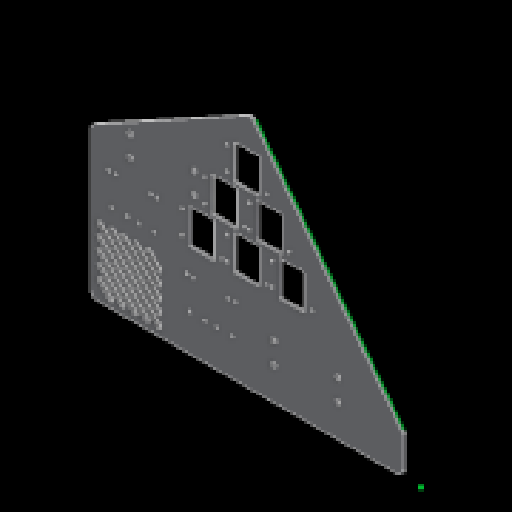
# Autodesk Inventor part: SideChestPanel
Saved by Autodesk Inventor 2025.2 (Build 292293000, 293)
## iProperties
Created: 2025-10-06
Part Number: SideChestPanel
Material: Generic
Document SubType Name: Sheet Metal
Designer: valer
Density: 1 g/cm^3
Sheet Metal Rule: Default
Appearance: Default
Author: valer
Autodesk Inventor part; units mm, degrees
note: some values were not read from the file. Chosen so that the rebuilt part matches the saved one: edges of "OutsideFilletsFeature".
ref_plane "YZ Plane" through (0, 0, 0) normal (1, 0, 0) x (0, 1, 0)
ref_plane "XZ Plane" through (0, 0, 0) normal (0, 1, 0) x (-1, 0, 0)
ref_plane "XY Plane" through (0, 0, 0) normal (0, 0, 1) x (1, 0, 0)
sketch "Base" plane through (0, 0, 0) normal (0, 0, 1) x (1, 0, 0)
  line L0 (-378.7052, 89.8796) -> (-378.7052, 174.3855)
  line L1 (-378.7052, 174.3855) -> (-195.1416, 275.4647)
  line L2 (-195.1416, 275.4647) -> (-175.6395, 271.0298)
  line L3 (-175.6395, 271.0298) -> (-18.7052, 51.3218)
  line L4 (-18.7052, 51.3218) -> (-18.7052, 2.2456)
  line L5 (-18.7052, 2.2456) -> (-378.7052, 2.2456)
  line L6 (-378.7052, 2.2456) -> (-378.7052, 89.8796)
  line L7 (-389.1847, 101.2829) -> (-389.1847, 49.3817) construction
  line L8 (-169.8355, 262.9042) -> (-11.397, 41.0903) construction
  line L9 (-372.782, 2.2456) -> (-8.9217, 2.2456) construction
  line L10 (-202.0962, 271.6351) -> (-397.656, 163.9503) construction
  point P0 (0, 0)
  dimension "d40" = 360
  dimension "d41" = 270
  dimension "d42" = 20
  dimension "d43" = 138.349
  dimension "d44" = 138.349
  measures "d40" distance of L4.end L5.end
  measures "d41" distance of L2.end L3.end
  measures "d42" distance of L1.end L2.end
  measures "d43" angle of L3 L2
  measures "d44" angle of L2 L1
extrude "Plate1" add sketch "Base" along normal blind 3
fillet "OutsideFilletsFeature" radius 6 5 edges at (-378.7052, 2.2456, 1.5) (-18.7052, 2.2456, 1.5) (-18.7052, 51.3218, 1.5) (-175.6395, 271.0298, 1.5) (-195.1416, 275.4647, 1.5)
sketch "HardwareMountHoles" plane through (0, 0, 0) normal (0, 0, -1) x (-1, 0, 0)
  circle A0 centre (175.3952, 206.6354) radius 1.5 projected
  circle A1 centre (221.3566, 233.1714) radius 1.5 projected
  circle A2 centre (149.4146, 161.6352) radius 1.5 projected
  circle A3 centre (195.3761, 161.6353) radius 1.5 projected
  circle A4 centre (195.3761, 188.1712) radius 1.5 projected
  circle A5 centre (221.3567, 206.6355) radius 1.5 projected
  circle A6 centre (201.3761, 161.6355) radius 1.5
  circle A7 centre (247.3376, 161.6357) radius 1.5
  circle A8 centre (247.3375, 188.1716) radius 1.5
  circle A9 centre (227.3571, 116.6357) radius 1.5
  circle A10 centre (273.3186, 116.6361) radius 1.5
  circle A11 centre (273.3184, 143.172) radius 1.5
  circle A12 centre (175.3956, 116.6353) radius 1.5
  circle A13 centre (221.3571, 116.6356) radius 1.5
  circle A14 centre (221.3569, 143.1715) radius 1.5
  circle A15 centre (123.4341, 116.635) radius 1.5
  circle A16 centre (169.3956, 116.6352) radius 1.5
  circle A17 centre (169.3954, 143.1711) radius 1.5
  circle A18 centre (123.4339, 143.1709) radius 1.5
  point P0 (0, 0)
  constraints: 13 centre point, 26 other
extrude "HardwareMountHolesFeature" cut sketch "HardwareMountHoles" against normal blind 3 contours A0 | A1 | A2 | A3 | A4 | A5 | A6 | A7 | A8 | A9 | A10 | A11 | A12 | A13 | A14 | A15 | A16 | A17
sketch "HeatsinkCut1" plane through (0, 0, 3) normal (0, 0, 1) x (1, 0, 0)
  line L0 (-185.8757, 238.2531) -> (-210.9757, 238.2534) projected
  line L1 (-185.876, 201.5531) -> (-185.8757, 238.2531) projected
  line L2 (-210.9757, 238.2534) -> (-210.976, 201.5534) projected
  line L3 (-210.976, 201.5534) -> (-185.876, 201.5531) projected
  point P0 (0, 0)
extrude "HeatsinkCut1Feature" cut sketch "HeatsinkCut1" against normal blind 3
sketch "HeatsinkCut2" plane through (0, 0, 3) normal (0, 0, 1) x (1, 0, 0)
  line L0 (-159.8953, 193.2532) -> (-184.9953, 193.2533) projected
  line L1 (-184.9953, 193.2533) -> (-184.9954, 156.5533) projected
  line L2 (-159.8954, 156.5532) -> (-159.8953, 193.2532) projected
  line L3 (-184.9954, 156.5533) -> (-159.8954, 156.5532) projected
  point P0 (0, 0)
extrude "HeatsinkCut2Feature" cut sketch "HeatsinkCut2" against normal blind 3
sketch "HeatsinkCut3" plane through (0, 0, 3) normal (0, 0, 1) x (1, 0, 0)
  line L0 (-211.8568, 193.2535) -> (-236.9568, 193.2536) projected
  line L1 (-211.8569, 156.5535) -> (-211.8568, 193.2535) projected
  line L2 (-236.9569, 156.5536) -> (-211.8569, 156.5535) projected
  line L3 (-236.9569, 156.5536) -> (-236.9568, 193.2536)
  point P0 (0, 0)
  constraints: 2 end point
extrude "HeatsinkCut3Feature" cut sketch "HeatsinkCut3" against normal blind 3
sketch "HeatsinkCut4" plane through (0, 0, 3) normal (0, 0, 1) x (1, 0, 0)
  line L0 (-237.8376, 148.2538) -> (-262.9376, 148.254) projected
  line L1 (-262.9376, 148.254) -> (-262.9379, 111.554) projected
  line L2 (-237.8379, 111.5538) -> (-237.8376, 148.2538) projected
  line L3 (-262.9379, 111.554) -> (-237.8379, 111.5538) projected
  point P0 (0, 0)
extrude "HeatsinkCut4Feature" cut sketch "HeatsinkCut4" against normal blind 3
sketch "HeatsinkCut5" plane through (0, 0, 3) normal (0, 0, 1) x (1, 0, 0)
  line L0 (-185.8761, 148.2534) -> (-210.9761, 148.2535) projected
  line L1 (-185.8764, 111.5534) -> (-185.8761, 148.2534) projected
  line L2 (-210.9764, 111.5535) -> (-185.8764, 111.5534) projected
  line L3 (-210.9761, 148.2535) -> (-210.9764, 111.5535) projected
  line L4 (-185.8761, 148.2534) -> (-210.9761, 148.2535) projected
  point P0 (0, 0)
extrude "HeatsinkCut5Feature" cut sketch "HeatsinkCut5" against normal blind 3
sketch "HeatsinkCut6" plane through (0, 0, 3) normal (0, 0, 1) x (1, 0, 0)
  line L0 (-133.9147, 148.253) -> (-159.0147, 148.2532) projected
  line L1 (-133.9148, 111.553) -> (-133.9147, 148.253) projected
  line L2 (-159.0147, 148.2532) -> (-159.0148, 111.5532) projected
  line L3 (-133.9147, 148.253) -> (-159.0147, 148.2532) projected
  line L4 (-159.0147, 148.2532) -> (-159.0148, 111.5532) projected
  line L5 (-159.0148, 111.5532) -> (-133.9148, 111.553) projected
  point P0 (0, 0)
extrude "HeatsinkCut6Feature" cut sketch "HeatsinkCut6" against normal blind 3
sketch "AdjustToProduction" plane through (0, 0, 3) normal (0, 0, 1) x (1, 0, 0)
  line L0 (-18.7052, 49.399) -> (-18.7052, 8.2456) projected
  line L1 (-18.7052, 46.0604) -> (-192.9162, 274.9586)
  line L2 (-174.313, 269.1727) -> (-19.8228, 52.8864) projected
  line L3 (-192.9162, 274.9586) -> (-177.8649, 271.5359) projected
  arc A0 (-174.313, 269.1727) -> (-177.8649, 271.5359) centre (-179.1954, 265.6852) ccw projected
  arc A1 (-18.7052, 49.399) -> (-19.8228, 52.8864) centre (-24.7052, 49.399) ccw projected
  point P0 (0, 0)
  constraints: 2 end point, 1 point on line
extrude "AdjustToProductionFeature" cut sketch "AdjustToProduction" against normal blind 3
delete faces "Delete1" heal yes whole lump no faces at (-196.2577, 274.7609, 1)
fillet "ProductionReFilletFeature" radius 6 3 edges at (-193.8448, 276.1787, 1.5) (-18.7052, 46.0604, 1.5) (-378.7052, 174.3855, 1.5)
sketch "WidenHeatsinkHoles" plane through (-372.7052, 2.2456, 3) normal (0, 0, 1) x (1, 0, 0)
  arc A0 (354, 41.7913) -> (352.7745, 45.425) centre (348, 41.7913) ccw projected
  line L0 (352.7745, 45.425) -> (181.995, 269.8145) projected
  arc A1 (181.995, 269.8145) -> (174.3264, 271.4366) centre (177.2206, 266.1807) ccw projected
  line L1 (-2.8941, 173.8502) -> (174.3264, 271.4366) projected
  line L2 (-6, 6) -> (-6, 168.5943) projected
  arc A2 (-6, 6) -> (0, 0) centre (0, 6) ccw projected
  line L3 (348, 0) -> (0, 0) projected
  arc A3 (348, 0) -> (354, 6) centre (348, 6) ccw projected
  line L4 (354, 41.7913) -> (354, 6) projected
  circle A4 centre (145.3481, 114.3902) radius 1.5 projected
  circle A5 centre (249.2711, 114.3895) radius 1.5 projected
  circle A6 centre (99.3868, 140.9265) radius 1.5 projected
  circle A7 centre (171.329, 159.39) radius 1.5 projected
  circle A8 centre (151.3485, 204.3899) radius 1.5 projected
  circle A9 centre (197.31, 204.3898) radius 1.5 projected
  circle A10 centre (151.3483, 140.926) radius 1.5 projected
  circle A11 centre (99.3866, 114.3906) radius 1.5 projected
  circle A12 centre (203.3096, 114.3897) radius 1.5 projected
  circle A13 centre (151.3481, 114.39) radius 1.5 projected
  circle A14 centre (223.2906, 159.3897) radius 1.5 projected
  circle A15 centre (125.3675, 159.3902) radius 1.5 projected
  circle A16 centre (177.3291, 159.3898) radius 1.5 projected
  circle A17 centre (151.3485, 230.9258) radius 1.5 projected
  circle A18 centre (177.3291, 185.9257) radius 1.5 projected
  circle A19 centre (125.3677, 185.9261) radius 1.5 projected
  circle A20 centre (203.3098, 140.9256) radius 1.5 projected
  circle A21 centre (197.3096, 114.3897) radius 1.5 projected
  line L5 (186.8292, 199.3076) -> (161.7292, 199.3078) projected
  line L6 (161.7292, 199.3078) -> (161.7295, 236.0078) projected
  line L7 (161.7295, 236.0078) -> (186.8295, 236.0076) projected
  line L8 (186.8295, 236.0076) -> (186.8292, 199.3076) projected
  line L9 (212.8098, 154.3077) -> (187.7098, 154.3077) projected
  line L10 (187.7098, 154.3077) -> (187.7099, 191.0077) projected
  line L11 (187.7099, 191.0077) -> (212.8099, 191.0077) projected
  line L12 (212.8099, 191.0077) -> (212.8098, 154.3077) projected
  line L13 (135.7484, 191.0081) -> (160.8484, 191.008) projected
  line L14 (160.8484, 191.008) -> (160.8483, 154.308) projected
  line L15 (160.8483, 154.308) -> (135.7483, 154.3081) projected
  line L16 (135.7483, 154.3081) -> (135.7484, 191.0081) projected
  line L17 (134.8673, 109.3082) -> (109.7673, 109.3084) projected
  line L18 (109.7673, 109.3084) -> (109.7676, 146.0084) projected
  line L19 (109.7676, 146.0084) -> (134.8676, 146.0082) projected
  line L20 (134.8676, 146.0082) -> (134.8673, 109.3082) projected
  line L21 (161.7288, 109.308) -> (161.7291, 146.008) projected
  line L22 (161.7291, 146.008) -> (186.8291, 146.0078) projected
  line L23 (186.8291, 146.0078) -> (186.8288, 109.3078) projected
  line L24 (186.8288, 109.3078) -> (161.7288, 109.308) projected
  line L25 (213.6904, 109.3076) -> (213.6905, 146.0076) projected
  line L26 (213.6905, 146.0076) -> (238.7905, 146.0075) projected
  line L27 (238.7905, 146.0075) -> (238.7904, 109.3075) projected
  line L28 (238.7904, 109.3075) -> (213.6904, 109.3076) projected
  line L29 (211.6904, 107.3076) -> (211.6905, 148.0076)
  line L30 (211.6905, 148.0076) -> (240.7905, 148.0075)
  line L31 (240.7905, 148.0075) -> (240.7904, 107.3075)
  line L32 (240.7904, 107.3075) -> (211.6904, 107.3076)
  line L33 (159.7288, 107.308) -> (159.7291, 148.008)
  line L34 (159.7291, 148.008) -> (188.8291, 148.0078)
  line L35 (188.8291, 148.0078) -> (188.8288, 107.3078)
  line L36 (188.8288, 107.3078) -> (159.7288, 107.308)
  line L37 (185.7098, 152.3077) -> (214.8098, 152.3077)
  line L38 (214.8098, 152.3077) -> (214.8099, 193.0077)
  line L39 (214.8099, 193.0077) -> (185.7099, 193.0077)
  line L40 (185.7099, 193.0077) -> (185.7098, 152.3077)
  line L41 (133.7483, 152.3081) -> (162.8483, 152.308)
  line L42 (162.8483, 152.308) -> (162.8484, 193.008)
  line L43 (162.8484, 193.008) -> (133.7484, 193.0081)
  line L44 (133.7484, 193.0081) -> (133.7483, 152.3081)
  line L45 (159.7292, 197.3078) -> (188.8292, 197.3076)
  line L46 (188.8292, 197.3076) -> (188.8295, 238.0076)
  line L47 (188.8295, 238.0076) -> (159.7295, 238.0078)
  line L48 (159.7295, 238.0078) -> (159.7292, 197.3078)
  line L49 (107.7673, 107.3085) -> (136.8673, 107.3082)
  line L50 (136.8673, 107.3082) -> (136.8676, 148.0082)
  line L51 (136.8676, 148.0082) -> (107.7676, 148.0085)
  line L52 (107.7676, 148.0085) -> (107.7673, 107.3085)
  arc A22 (-2.8941, 173.8502) -> (-6, 168.5943) centre (0, 168.5943) ccw projected
  point P0 (372.7052, -2.2456)
  dimension "d56" = 2
  dimension "d57" = 2
  dimension "d58" = 2
  dimension "d59" = 2
  dimension "d60" = 2
  dimension "d61" = 2
  constraints: 48 end point, 18 other
  measures "d56" distance between parallel lines of L28 L32
  measures "d57" distance between parallel lines of L24 L36
  measures "d58" distance between parallel lines of L9 L37
  measures "d59" distance between parallel lines of L15 L41
  measures "d60" distance between parallel lines of L5 L45
  measures "d61" distance between parallel lines of L17 L49
extrude "WidenHeatsinkHolesFeature" cut sketch "WidenHeatsinkHoles" against normal blind 3 contours L5 L6 L7 L8 | L9 L10 L11 L12 | L13 L14 L15 L16 | L17 L18 L19 L20 | L21 L22 L23 L24 | L25 L26 L27 L28 | L29 L30 L31 L32 | L33 L34 L35 L36 | L40 L39 L38 L37 | L44 L43 L42 L41 | L48 L47 L46 L45 | L52 L51 L50 L49
fillet "HeatsinkHoleFilletsFeature" radius 1 24 edges at (-264.9379, 109.554, 1.5) (-235.8379, 109.5538, 1.5) (-235.8376, 150.2538, 1.5) (-264.9376, 150.254, 1.5) (-212.9764, 109.5535, 1.5) (-183.8764, 109.5533, 1.5) (-183.8761, 150.2533, 1.5) (-212.9761, 150.2535, 1.5) (-209.8569, 154.5535, 1.5) (-238.9569, 154.5537, 1.5) (-238.9568, 195.2537, 1.5) (-209.8568, 195.2535, 1.5) (-186.9954, 154.5533, 1.5) (-157.8954, 154.5532, 1.5) (-186.9953, 195.2533, 1.5) (-157.8953, 195.2532, 1.5) (-161.0148, 109.5532, 1.5) (-131.9148, 109.553, 1.5) (-131.9147, 150.253, 1.5) (-161.0147, 150.2532, 1.5) (-212.976, 199.5534, 1.5) (-183.876, 199.5531, 1.5) (-183.8757, 240.2531, 1.5) (-212.9757, 240.2534, 1.5)
sketch "MountHoles1" plane through (-24.7052, 2.2456, 0) normal (0, 0, -1) x (-1, 0, 0)
  circle A0 centre (68.5, 38) radius 3
  circle A1 centre (68.5, 62) radius 3
  circle A2 centre (142.5, 62) radius 3
  circle A3 centre (142.5, 38) radius 3
  circle A4 centre (190.5, 42.5) radius 1.6
  circle A5 centre (222, 42.5) radius 1.6
  circle A6 centre (235.5, 78.42) radius 1.6
  circle A7 centre (187.0915, 78.5) radius 1.6
  circle A8 centre (308.6323, 185.9084) radius 3
  circle A9 centre (308.6324, 161.9084) radius 3
  circle A10 centre (234.6323, 185.9081) radius 3
  circle A11 centre (234.6324, 161.9081) radius 3
  circle A12 centre (311.8137, 101.5) radius 1.6
  circle A13 centre (280.3137, 101.5) radius 1.6
  circle A14 centre (276.9052, 137.5) radius 1.6
  circle A15 centre (325.3137, 137.42) radius 1.6
  point P0 (-24.7052, -2.2456)
  point P1 (300.7283, 191.2583)
  constraints: 16 centre point, 33 other
extrude "MountHoles1Feature" cut sketch "MountHoles1" against normal blind 3
sketch "MountHoles2" plane through (-372.7052, 2.2456, 3) normal (0, 0, 1) x (1, 0, 0)
  circle A0 centre (139.5, 42.5) radius 1.6
  circle A1 centre (108, 42.5) radius 1.6
  circle A2 centre (104.5915, 78.5) radius 1.6
  circle A3 centre (153, 78.42) radius 1.6
  circle A4 centre (49.6863, 101.5) radius 1.6
  circle A5 centre (18.1863, 101.5) radius 1.6
  circle A6 centre (14.7778, 137.5) radius 1.6
  circle A7 centre (63.1863, 137.42) radius 1.6
  point P0 (372.7052, -2.2456)
  constraints: 8 centre point, 16 other
extrude "MountHoles2Feature" cut sketch "MountHoles2" against normal blind 3
sketch "FrontVentHoles" plane through (-24.7052, 2.2456, 0) normal (0, 0, -1) x (-1, 0, 0)
  line L0 (344, 10) -> (269, 10) construction
  line L1 (269, 10) -> (269, 79) construction
  line L2 (269, 79) -> (344, 79) construction
  line L3 (344, 79) -> (344, 10) construction
  line L4 (348, 0) -> (0, 0) projected
  line L5 (354, 168.5943) -> (354, 6) projected
  line L6 (259, 82.5) -> (259, 32.5) construction
  line L7 (346.3137, 89) -> (263.8137, 89) construction
  line L8 (344, 22.7279) -> (331.2721, 10) construction
  line L9 (341.8787, 24.8492) -> (329.1508, 12.1213)
  line L10 (333.3934, 7.8787) -> (346.1213, 20.6066)
  arc A0 (346.1213, 20.6066) -> (341.8787, 24.8492) centre (344, 22.7279) ccw
  arc A1 (329.1508, 12.1213) -> (333.3934, 7.8787) centre (331.2721, 10) ccw
  line L11 (344, 36.8701) -> (317.1299, 10) construction
  line L12 (346.1213, 34.7487) -> (319.2513, 7.8787)
  line L13 (315.0086, 12.1213) -> (341.8787, 38.9914)
  arc A2 (346.1213, 34.7487) -> (341.8787, 38.9914) centre (344, 36.8701) ccw
  arc A3 (315.0086, 12.1213) -> (319.2513, 7.8787) centre (317.1299, 10) ccw
  line L14 (344, 51.0122) -> (302.9878, 10) construction
  line L15 (346.1213, 48.8909) -> (305.1091, 7.8787)
  line L16 (300.8665, 12.1213) -> (341.8787, 53.1335)
  arc A4 (346.1213, 48.8909) -> (341.8787, 53.1335) centre (344, 51.0122) ccw
  arc A5 (300.8665, 12.1213) -> (305.1091, 7.8787) centre (302.9878, 10) ccw
  line L17 (344, 65.1543) -> (288.8457, 10) construction
  line L18 (346.1213, 63.033) -> (290.967, 7.8787)
  line L19 (286.7244, 12.1213) -> (341.8787, 67.2756)
  arc A6 (346.1213, 63.033) -> (341.8787, 67.2756) centre (344, 65.1543) ccw
  arc A7 (286.7244, 12.1213) -> (290.967, 7.8787) centre (288.8457, 10) ccw
  line L20 (274.7035, 10) -> (343.7035, 79) construction
  line L21 (272.5822, 12.1213) -> (341.5822, 81.1213)
  line L22 (345.8249, 76.8787) -> (276.8249, 7.8787)
  arc A8 (272.5822, 12.1213) -> (276.8249, 7.8787) centre (274.7035, 10) ccw
  arc A9 (345.8249, 76.8787) -> (341.5822, 81.1213) centre (343.7035, 79) ccw
  line L23 (343.7035, 79.2965) -> (274.7035, 79.2965) construction
  line L24 (289.5528, 77.1751) -> (276.8249, 64.4472)
  line L25 (272.5822, 68.6899) -> (285.3101, 81.4178)
  arc A10 (289.5528, 77.1751) -> (285.3101, 81.4178) centre (287.4315, 79.2965) ccw
  arc A11 (272.5822, 68.6899) -> (276.8249, 64.4472) centre (274.7035, 66.5685) ccw
  line L26 (299.4523, 81.4178) -> (272.5822, 54.5477)
  line L27 (276.8249, 50.3051) -> (303.6949, 77.1751)
  arc A12 (303.6949, 77.1751) -> (299.4523, 81.4178) centre (301.5736, 79.2965) ccw
  arc A13 (272.5822, 54.5477) -> (276.8249, 50.3051) centre (274.7035, 52.4264) ccw
  line L28 (313.5944, 81.4178) -> (272.5822, 40.4056)
  line L29 (276.8249, 36.163) -> (317.837, 77.1751)
  arc A14 (317.837, 77.1751) -> (313.5944, 81.4178) centre (315.7157, 79.2965) ccw
  arc A15 (272.5822, 40.4056) -> (276.8249, 36.163) centre (274.7035, 38.2843) ccw
  line L30 (329.8579, 79.2965) -> (274.7035, 24.1421) construction
  line L31 (327.7365, 81.4178) -> (272.5822, 26.2635)
  line L32 (276.8249, 22.0208) -> (331.9792, 77.1751)
  arc A16 (331.9792, 77.1751) -> (327.7365, 81.4178) centre (329.8579, 79.2965) ccw
  arc A17 (272.5822, 26.2635) -> (276.8249, 22.0208) centre (274.7035, 24.1421) ccw
  point P0 (-24.7052, -2.2456)
  point P1 (337.636, 16.364)
  point P2 (330.565, 23.435)
  point P3 (323.4939, 30.5061)
  point P4 (316.4228, 37.5772)
  point P5 (309.2035, 44.5)
  dimension "d86" = 10
  dimension "d87" = 10
  dimension "d88" = 10
  dimension "d89" = 10
  dimension "d90" = 3
  dimension "d91" = 45
  dimension "d92" = 18
  dimension "d93" = 10
  dimension "d94" = 10
  dimension "d95" = 10
  dimension "d96" = 10
  constraints: 74 end point, 36 point on circle, 26 symmetric about line, 20 tangent, 18 centre point, 14 point on line, 11 parallel, 5 midpoint, 4 equal radius, 2 horizontal, 1 perpendicular, 1 vertical, 12 other
  measures "d86" distance between parallel lines of L4 L0
  measures "d87" distance between parallel lines of L5 L3
  measures "d88" distance between parallel lines of L6 L1
  measures "d89" distance between parallel lines of L7 L2
  measures "d90" radius of A1
  measures "d91" angle of L0 L8
  measures "d92" distance of L8.start L8.end
  measures "d93" distance between parallel lines of L11 L8
  measures "d94" distance between parallel lines of L14 L11
  measures "d95" distance between parallel lines of L17 L14
  measures "d96" distance between parallel lines of L20 L17
extrude "FrontVentHolesFeature" cut sketch "FrontVentHoles" against normal blind 3
sketch "BackVentHoles" plane through (-24.7052, 2.2456, 0) normal (0, 0, -1) x (-1, 0, 0)
  line L0 (58.5, 10) -> (4, 10) construction
  line L1 (4, 10) -> (4, 40.4422) construction
  line L2 (4, 40.4422) -> (58.5, 112.0505) construction
  line L3 (58.5, 112.0505) -> (58.5, 10) construction
  line L4 (348, 0) -> (0, 0) projected
  line L5 (166.005, 269.8145) -> (-4.7745, 45.425) projected
  line L6 (-6, 6) -> (-6, 41.7913) projected
  circle A0 centre (68.5, 38) radius 3 projected
  line L7 (8.2426, 10) -> (4, 14.2426) construction
  line L8 (6.1213, 7.8787) -> (1.8787, 12.1213)
  line L9 (6.1213, 16.364) -> (10.364, 12.1213)
  arc A1 (6.1213, 7.8787) -> (10.364, 12.1213) centre (8.2426, 10) ccw
  arc A2 (6.1213, 16.364) -> (1.8787, 12.1213) centre (4, 14.2426) ccw
  line L10 (22.3848, 10) -> (4, 28.3848) construction
  line L11 (20.2635, 7.8787) -> (1.8787, 26.2635)
  line L12 (6.1213, 30.5061) -> (24.5061, 12.1213)
  arc A3 (20.2635, 7.8787) -> (24.5061, 12.1213) centre (22.3848, 10) ccw
  arc A4 (6.1213, 30.5061) -> (1.8787, 26.2635) centre (4, 28.3848) ccw
  line L13 (4.9009, 41.626) -> (36.5269, 10) construction
  line L14 (7.0223, 43.7473) -> (38.6482, 12.1213)
  line L15 (34.4056, 7.8787) -> (2.7796, 39.5047)
  arc A5 (7.0223, 43.7473) -> (2.7796, 39.5047) centre (4.9009, 41.626) ccw
  arc A6 (34.4056, 7.8787) -> (38.6482, 12.1213) centre (36.5269, 10) ccw
  arc A7 (272.5822, 12.1213) -> (276.8249, 7.8787) centre (274.7035, 10) ccw projected
  line L16 (50.669, 10) -> (11.0127, 49.6563) construction
  line L17 (52.7904, 12.1213) -> (13.134, 51.7777)
  line L18 (8.8914, 47.535) -> (48.5477, 7.8787)
  arc A8 (48.5477, 7.8787) -> (52.7904, 12.1213) centre (50.669, 10) ccw
  arc A9 (13.134, 51.7777) -> (8.8914, 47.535) centre (11.0127, 49.6563) ccw
  line L19 (58.5, 16.3112) -> (17.1245, 57.6867) construction
  line L20 (56.3787, 14.1899) -> (15.0032, 55.5654)
  line L21 (19.2458, 59.808) -> (60.6213, 18.4325)
  arc A10 (56.3787, 14.1899) -> (60.6213, 18.4325) centre (58.5, 16.3112) ccw
  arc A11 (19.2458, 59.808) -> (15.0032, 55.5654) centre (17.1245, 57.6867) ccw
  point P0 (-24.7052, -2.2456)
  point P1 (6.1213, 12.1213)
  point P2 (13.1924, 19.1924)
  point P3 (20.7139, 25.813)
  point P4 (30.8409, 29.8282)
  point P5 (37.8122, 36.9989)
  dimension "d99" = 10
  dimension "d100" = 10
  dimension "d101" = 10
  dimension "d102" = 10
  dimension "d103" = 45
  dimension "d104" = 10
  dimension "d105" = 10
  dimension "d106" = 6
  dimension "d107" = 10
  dimension "d108" = 10
  constraints: 48 end point, 20 point on circle, 20 tangent, 11 parallel, 10 centre point, 10 point on line, 5 equal radius, 5 midpoint, 2 perpendicular, 1 horizontal
  measures "d99" distance between parallel lines of L4 L0
  measures "d100" distance between parallel lines of L6 L1
  measures "d101" distance between parallel lines of L5 L2
  measures "d102" distance from line of A0.centre L3
  measures "d103" angle of L0 L7
  measures "d104" distance between parallel lines of L10 L7
  measures "d105" distance between parallel lines of L13 L10
  measures "d106" distance of L7.start L7.end
  measures "d107" distance between parallel lines of L16 L13
  measures "d108" distance between parallel lines of L19 L16
extrude "BackVentHolesFeature" cut sketch "BackVentHoles" against normal blind 3 contours L8 A2 L9 A1 | L11 A4 L12 A3 | L14 A6 L15 A5 | A8 L18 A9 L17 | L20 A11 L21 A10
sketch "ArmBoardVents" plane through (-24.7052, 2.2456, 0) normal (0, 0, -1) x (-1, 0, 0)
  line L0 (282.7778, 109) -> (266.7778, 130)
  line L1 (266.7778, 130) -> (298.7778, 130)
  line L2 (298.7778, 130) -> (282.7778, 109)
  line L3 (289.0637, 109) -> (305.0637, 130)
  line L4 (305.0637, 130) -> (321.0637, 109)
  line L5 (321.0637, 109) -> (289.0637, 109)
  line L6 (346.3137, 89) -> (263.8137, 89) construction
  line L7 (263.8137, 144) -> (346.3137, 144) construction
  line L8 (305.0637, 89) -> (305.0637, 144) construction
  line L9 (289.0637, 109) -> (282.7778, 109) construction
  line L10 (305.0637, 130) -> (298.7778, 130) construction
  circle A0 centre (276.9052, 137.5) radius 1.6 projected
  circle A1 centre (280.3137, 101.5) radius 1.6 projected
  line L11 (327.3496, 109) -> (343.3496, 130)
  line L12 (343.3496, 130) -> (311.3496, 130)
  line L13 (311.3496, 130) -> (327.3496, 109)
  line L14 (256.5, 30) -> (174, 30) construction
  line L15 (174, 85) -> (256.5, 85) construction
  line L16 (215.25, 30) -> (215.25, 85) construction
  line L17 (231.25, 50) -> (199.25, 50)
  line L18 (199.25, 50) -> (215.25, 71)
  line L19 (231.25, 50) -> (215.25, 71)
  line L20 (208.9641, 71) -> (192.9641, 50)
  line L21 (192.9641, 50) -> (176.9641, 71)
  line L22 (176.9641, 71) -> (208.9641, 71)
  line L23 (215.25, 71) -> (208.9641, 71) construction
  line L24 (199.25, 50) -> (192.9641, 50) construction
  line L25 (221.5359, 71) -> (237.5359, 50)
  line L26 (237.5359, 50) -> (253.5359, 71)
  line L27 (253.5359, 71) -> (221.5359, 71)
  point P0 (-24.7052, -2.2456)
  point P1 (305.0637, 109)
  dimension "d111" = 32
  dimension "d112" = 5
  dimension "d113" = 14
  dimension "d114" = 7.5
  dimension "d115" = 7.5
  dimension "d116" = 14
  dimension "d117" = 20
  dimension "d118" = 20
  dimension "d119" = 5
  constraints: 56 end point, 9 horizontal, 6 symmetric about line, 5 equal length, 5 midpoint, 3 point on line, 2 collinear, 1 parallel, 1 perpendicular, 8 other
  measures "d111" distance of L0.end L1.end
  measures "d112" distance between parallel lines of L2 L3
  measures "d113" distance between parallel lines of L7 L1
  measures "d114" distance from line of A0.centre L1
  measures "d115" distance from line of L9 A1.centre
  measures "d116" distance from line of L15 L18.end
  measures "d117" distance between parallel lines of L6 L5
  measures "d118" distance between parallel lines of L14 L17
  measures "d119" distance between parallel lines of L18 L20
extrude "ArmBoardVentsFeature" cut sketch "ArmBoardVents" against normal blind 3 contours L0 L1 L2 | L3 L4 L5 | L13 L12 L11 | L17 L18 L19 | L20 L21 L22 | L27 L26 L25
fillet "ArmBoardVentsFilletsFeature" radius 2 18 edges at (-352.0548, 111.2456, 1.5) (-368.0548, 132.2456, 1.5) (-336.0548, 132.2456, 1.5) (-345.7689, 111.2456, 1.5) (-329.7689, 132.2456, 1.5) (-313.7689, 111.2456, 1.5) (-307.483, 111.2456, 1.5) (-323.483, 132.2456, 1.5) (-291.483, 132.2456, 1.5) (-278.2411, 73.2456, 1.5) (-262.2411, 52.2456, 1.5) (-246.2411, 73.2456, 1.5) (-255.9552, 52.2456, 1.5) (-223.9552, 52.2456, 1.5) (-239.9552, 73.2456, 1.5) (-233.6693, 73.2456, 1.5) (-217.6693, 52.2456, 1.5) (-201.6693, 73.2456, 1.5)
equation "\"d43\" = d44"
equation "\"d24\" = Thickness"
equation "\"d28\" = Thickness"
equation "\"d30\" = Thickness"
equation "\"d32\" = Thickness"
equation "\"d34\" = Thickness"
equation "\"d36\" = Thickness"
equation "\"d38\" = Thickness"
equation "\"d53\" = Thickness"
equation "\"d62\" = Thickness"
equation "\"d67\" = Thickness"
equation "\"d69\" = Thickness"
equation "\"d0\" = Thickness"
equation "\"BendRadius\" = Thickness"
equation "\"BendReliefWidth\" = Thickness"
equation "\"BendReliefDepth\" = 0.5 * Thickness"
equation "\"CornerReliefSize\" = 4 * Thickness"
equation "\"MinimumRemnant\" = 2 * Thickness"
equation "\"TransitionRadius\" = BendRadius"
equation "\"JacobiRadiusSize\" = BendRadius"
equation "\"GapSize\" = Thickness"
equation "\"Thickness\" = 3"
body "Solid1"
